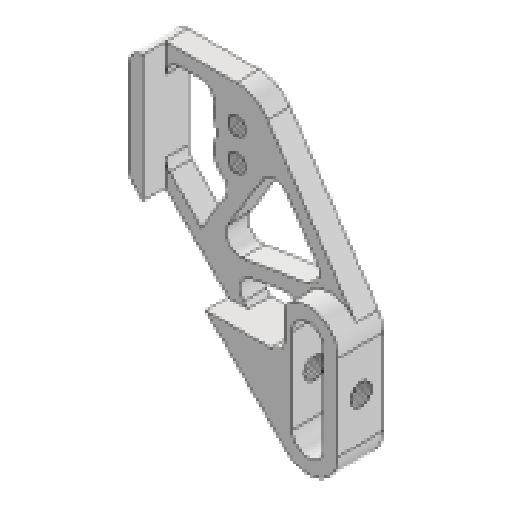
# Autodesk Inventor part: VerticalSlideMiddleBottom2.2
Saved by Autodesk Inventor 2023 (Build 270158000, 158)
## iProperties
Created: 2022-10-14
Part Number: VerticalSlideMiddleBottom2.2
Material: Generic
Document SubType Name: Modeling
Designer: deli
Density: 1 g/cm^3
Appearance: Default
Mass: 1.74743 g
Surface Area: 22.1752 cm^2
Volume: 1.74743 cm^3
Author: deli
Autodesk Inventor part; units mm, degrees
ref_plane "YZ Plane" through (0, 0, 0) normal (1, 0, 0) x (0, 1, 0)
ref_plane "XZ Plane" through (0, 0, 0) normal (0, 1, 0) x (-1, 0, 0)
ref_plane "XY Plane" through (0, 0, 0) normal (0, 0, 1) x (1, 0, 0)
sketch "Sketch1" plane through (0, 0, 0) normal (0, 0, 1) x (1, 0, 0)
  line L0 (-75.1619, -157.0247) -> (-75.1619, -170.0247)
  line L1 (-74.5821, -171.4329) -> (-52.9297, -193.2673)
  circle A0 centre (-63.1619, -164.7747) radius 1.25
  circle A1 centre (-63.1619, -160.2747) radius 1.25
  arc A2 (-52.1619, -190.2747) -> (-47.6619, -190.2747) centre (-49.9119, -190.2747) ccw
  arc A3 (-47.6619, -178.2747) -> (-52.1619, -178.2747) centre (-49.9119, -178.2747) ccw
  line L2 (-47.6619, -178.2747) -> (-47.6619, -190.2747)
  line L3 (-52.1619, -178.2747) -> (-52.1619, -190.2747)
  line L4 (-45.6619, -178.2747) -> (-45.6619, -190.2747)
  arc A4 (-52.9297, -193.2673) -> (-45.6619, -190.2747) centre (-49.9119, -190.2747) ccw
  arc A5 (-45.6619, -178.2747) -> (-46.38, -175.9108) centre (-49.9119, -178.2747) ccw
  line L5 (-46.38, -175.9108) -> (-58.7989, -157.3547)
  line L6 (-73.1619, -155.0247) -> (-63.1619, -155.0247)
  arc A6 (-58.7989, -157.3547) -> (-63.1619, -155.0247) centre (-63.1619, -160.2747) ccw
  arc A7 (-73.1619, -155.0247) -> (-75.1619, -157.0247) centre (-73.1619, -157.0247) ccw
  arc A8 (-75.1619, -170.0247) -> (-74.5821, -171.4329) centre (-73.1619, -170.0247) ccw
  line L7 (-52.1619, -182.7747) -> (-56.1619, -182.7747)
  line L8 (-56.1619, -182.7747) -> (-56.1619, -185.7747)
  line L9 (-56.1619, -185.7747) -> (-52.1619, -185.7747)
  point P0 (0, 0)
  dimension "d2" = 2.5
  dimension "d11" = 2
  dimension "d22" = 12
  dimension "d46" = 2
  dimension "d47" = 4.5
  dimension "d84" = 4
  dimension "d86" = 12
  dimension "d87" = 12
  dimension "d88" = 23
  dimension "d90" = 4
  dimension "d91" = 3
  dimension "d92" = 4.5
  dimension "d94" = 15
  dimension "d95" = 13.5
  dimension "d96" = 2
  constraints: 20 end point, 16 point on circle, 13 tangent, 9 centre point, 4 equal radius, 4 point on line, 3 perpendicular, 2 coincident, 2 vertical, 1 concentric, 1 horizontal, 1 parallel
  measures "d2" diameter of A0
  measures "d22" distance of A2.centre A3.centre
  measures "d46" radial gap between concentric circles of A4 A2
  measures "d47" distance between parallel lines of L2 L3
  measures "d84" distance edge to line of A1 L6
  measures "d86" distance from line of A1.centre L0
  measures "d87" distance from line of A0.centre L0
  measures "d88" distance between parallel lines of L3 L0
  measures "d90" distance of L7.start L7.end
  measures "d91" distance of L7.end L8.end
  measures "d92" distance from line of L3.start L7
  measures "d94" distance from line of L6 L0.end
  measures "d95" vertical distance of A3.centre A0.centre
  measures "d96" radius of A7
extrude "Extrusion1" add sketch "Sketch1" along normal blind 6.35 contours A7 L6 A6 L5 A5 L4 A4 L1 A8 L0 | L9 L8 L7 L3
thread "Thread2" size "M3x0.5" class "6H" standard "ANSI Metric M Profile" full length
thread "Thread6" size "M3x0.5" class "6H" standard "ANSI Metric M Profile" full length
sketch "Sketch8" plane through (-52.1619, -190.2747, 0) normal (1, 0, 0) x (0, 0, -1)
  line L0 (0, 0) -> (0, 12) construction
  line L1 (0, 12) -> (-6.35, 12) construction
  line L2 (-6.35, 0) -> (-6.35, 12) construction
  line L3 (0, 0) -> (-6.35, 0) construction
  line L4 (0, 0) -> (-6.35, 0) construction
  line L5 (-6.35, 12) -> (0, 0) construction
  line L6 (-6.35, 0) -> (0, 12) construction
  circle A0 centre (-3.175, 6) radius 1.5
  point P0 (0, 190.2747)
  dimension "d97" = 3
  constraints: 4 end point, 1 centre point, 1 midpoint
  measures "d97" diameter of A0
extrude "Extrusion7" cut sketch "Sketch8" along normal blind 10 and the other way blind 4
sketch "Sketch12" plane through (0, 0, 6.35) normal (0, 0, 1) x (1, 0, 0)
  line L0 (-75.1619, -157.0247) -> (-75.1619, -170.0247) projected
  arc A0 (-75.1619, -170.0247) -> (-74.5821, -171.4329) centre (-73.1619, -170.0247) ccw projected
  line L1 (-74.5821, -171.4329) -> (-52.9297, -193.2673) projected
  arc A1 (-52.9297, -193.2673) -> (-45.6619, -190.2747) centre (-49.9119, -190.2747) ccw projected
  line L2 (-45.6619, -190.2747) -> (-45.6619, -178.2747) projected
  arc A2 (-45.6619, -178.2747) -> (-46.38, -175.9108) centre (-49.9119, -178.2747) ccw projected
  line L3 (-46.38, -175.9108) -> (-58.7989, -157.3547) projected
  arc A3 (-58.7989, -157.3547) -> (-63.1619, -155.0247) centre (-63.1619, -160.2747) ccw projected
  line L4 (-63.1619, -155.0247) -> (-73.1619, -155.0247) projected
  arc A4 (-73.1619, -155.0247) -> (-75.1619, -157.0247) centre (-73.1619, -157.0247) ccw projected
  circle A5 centre (-63.1619, -164.7747) radius 1.25 projected
  circle A6 centre (-63.1619, -160.2747) radius 1.25 projected
  line L5 (-47.6619, -178.2747) -> (-47.6619, -190.2747) projected
  arc A7 (-52.1619, -190.2747) -> (-47.6619, -190.2747) centre (-49.9119, -190.2747) ccw projected
  line L6 (-52.1619, -190.2747) -> (-52.1619, -178.2747) projected
  arc A8 (-47.6619, -178.2747) -> (-52.1619, -178.2747) centre (-49.9119, -178.2747) ccw projected
  line L7 (-60.461, -158.467) -> (-50.0475, -174.0268)
  line L8 (-54.1619, -189.1843) -> (-73.1619, -170.0247)
  line L9 (-73.1619, -170.0247) -> (-73.1619, -157.0247)
  line L10 (-73.1619, -157.0247) -> (-63.1619, -157.0247)
  arc A9 (-65.5072, -162.5247) -> (-60.8167, -162.5247) centre (-63.1619, -164.7747) ccw
  line L11 (-54.1619, -178.2747) -> (-54.1619, -189.1843)
  arc A10 (-63.1619, -157.0247) -> (-65.5072, -162.5247) centre (-63.1619, -160.2747) ccw
  arc A11 (-60.8167, -162.5247) -> (-60.461, -158.467) centre (-63.1619, -160.2747) ccw
  arc A12 (-50.0475, -174.0268) -> (-54.1619, -178.2747) centre (-49.9119, -178.2747) ccw
  line L12 (-52.1619, -181.7747) -> (-61.5099, -181.7747)
  line L13 (-66.6094, -176.6323) -> (-57.865, -162.346)
  line L14 (-66.6094, -176.6323) -> (-50.0681, -173.9959)
  line L15 (-63.662, -167.986) -> (-68.0593, -175.1702)
  line L16 (-64.8751, -178.3812) -> (-53.8267, -176.6202)
  point P0 (0, 0)
  point P1 (-71.9729, -171.2237)
  point P2 (-56.8306, -163.8915)
  point P3 (-59.8632, -183.4351)
  point P4 (-58.2371, -185.0749)
  point P5 (-55.3555, -166.0957)
  point P6 (-73.1619, -163.7316)
  point P7 (-59.4375, -181.7747)
  point P8 (-54.1619, -181.7747)
  dimension "d108" = 2
  dimension "d110" = 2
  dimension "d111" = 2
  dimension "d112" = 2
  dimension "d113" = 2
  dimension "d114" = 2
  dimension "d115" = 2
  dimension "d116" = 2
  dimension "d124" = 3.5
  dimension "d134" = 2
  dimension "d135" = 2
  constraints: 19 end point, 10 point on circle, 6 point on line, 4 centre point, 2 parallel, 2 tangent, 1 equal length, 1 horizontal, 11 other
  measures "d108" distance between parallel lines of L3 L7
  measures "d110" radial gap between concentric circles of A5 A9
  measures "d111" distance between parallel lines of L6 L11
  measures "d112" radial gap between concentric circles of A6 A10
  measures "d113" radial gap between concentric circles of A6 A11
  measures "d114" radial gap between concentric circles of A8 A12
  measures "d116" distance between parallel lines of L0 L9
  measures "d124" distance from line of A2.centre L12
  measures "d134" distance between parallel lines of L13 L15
  measures "d135" distance between parallel lines of L14 L16
extrude "Extrusion10" cut sketch "Sketch12" against normal blind 10 contours L12 L8 L16 A12 L11 | L14 L13 L7 | L8 L9 L10 A10 A9 L15
fillet "Fillet6" radius 2 11 edges at (-73.1619, -157.0247, 3.175) (-63.1619, -157.0247, 3.175) (-65.5072, -162.5247, 3.175) (-54.1619, -181.7747, 3.175) (-73.1619, -170.0247, 3.175) (-63.662, -167.986, 3.175) (-50.0681, -173.9959, 3.175) (-66.6094, -176.6323, 3.175) (-57.865, -162.346, 3.175) (-53.8267, -176.6202, 3.175) (-64.8751, -178.3812, 3.175)
thread "Thread7" size "M3x0.5" class "6H" standard "ANSI Metric M Profile" full length
sketch "Sketch17" plane through (0, 0, 6.35) normal (0, 0, 1) x (1, 0, 0)
  line L0 (-73.1619, -147.1791) -> (-53.1619, -147.1791)
  line L1 (-53.1619, -147.1791) -> (-53.1619, -181.7747)
  line L2 (-53.1619, -181.7747) -> (-73.1619, -181.7747)
  line L3 (-73.1619, -181.7747) -> (-73.1619, -147.1791)
  line L4 (-75.1619, -157.0247) -> (-75.1619, -170.0247) projected
  line L5 (-52.1619, -190.2747) -> (-52.1619, -178.2747) projected
  line L6 (-56.1619, -181.7747) -> (-61.5099, -181.7747) projected
  arc A0 (-47.6619, -178.2747) -> (-52.1619, -178.2747) centre (-49.9119, -178.2747) ccw projected
  circle A1 centre (-49.9119, -178.2747) radius 4.25
  line L7 (-46.38, -175.9108) -> (-58.7989, -157.3547) projected
  point P0 (0, 0)
  point P1 (-53.1619, -175.5361)
  point P2 (-53.1619, -165.7773)
  dimension "d143" = 2
  dimension "d144" = 1
  constraints: 8 end point, 2 parallel, 1 coincident, 1 collinear, 1 horizontal, 1 perpendicular, 2 other
  measures "d143" distance between parallel lines of L4 L3
  measures "d144" distance between parallel lines of L5 L1
extrude "Extrusion14" cut sketch "Sketch17" against normal blind 3.175 contours L0 L1 A1 L2 L3 | L7 A1 L1 | L1 A1 picked at (-53.3437, -178.9123)
fillet "Fillet9" radius 2 2 edges at (-53.1619, -175.5361, 4.7625) (-53.1619, -181.7747, 4.7625)
equation "\"d22\" = d17"
equation "\"d17\" = 12"
body "Solid1"
